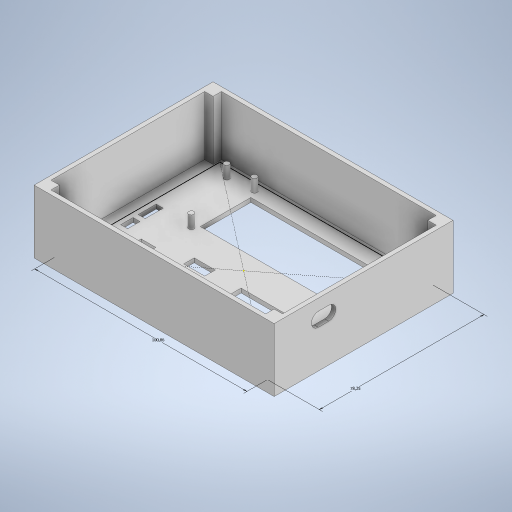
# Autodesk Inventor part: plant watner 2.0 case
Saved by Autodesk Inventor 2024 (Build 280153000, 153)
## iProperties
Created: 2024-03-16
Part Number: plant watner 2.0 case
Material: Generic
Document SubType Name: Modeling
Designer: Emil
Density: 1 g/cm^3
Appearance: Default
Author: Emil
Autodesk Inventor part; units mm, degrees
ref_plane "YZ Plane" through (0, 0, 0) normal (1, 0, 0) x (0, 1, 0)
ref_plane "XZ Plane" through (0, 0, 0) normal (0, 1, 0) x (-1, 0, 0)
ref_plane "XY Plane" through (0, 0, 0) normal (0, 0, 1) x (1, 0, 0)
sketch "Sketch1" plane through (0, 0, 0) normal (0, 1, 0) x (-1, 0, 0)
  line L0 (55, -40.5) -> (-55, -40.5)
  line L1 (-55, -40.5) -> (-55, 40.5)
  line L2 (-55, 40.5) -> (55, 40.5)
  line L3 (55, 40.5) -> (55, -40.5)
  line L4 (55, -40.5) -> (-55, 40.5) construction
  line L5 (-55, -40.5) -> (55, 40.5) construction
  line L6 (57, 42.5) -> (-57, 42.5)
  line L7 (-57, 42.5) -> (-57, -42.5)
  line L8 (-57, -42.5) -> (57, -42.5)
  line L9 (57, -42.5) -> (57, 42.5)
  line L10 (57, 42.5) -> (-57, -42.5) construction
  line L11 (-57, 42.5) -> (57, -42.5) construction
  line L12 (50.43, 39.125) -> (-50.43, 39.125)
  line L13 (-50.43, 39.125) -> (-50.43, -39.125)
  line L14 (-50.43, -39.125) -> (50.43, -39.125)
  line L15 (50.43, -39.125) -> (50.43, 39.125)
  line L16 (50.43, 39.125) -> (-50.43, -39.125) construction
  line L17 (-50.43, 39.125) -> (50.43, -39.125) construction
  point P0 (0, 0)
  dimension "d0" = 110
  dimension "d1" = 81
  dimension "d2" = 114
  dimension "d3" = 85
  dimension "d190" = 100.86
  dimension "d191" = 78.25
  constraints: 36 end point, 6 midpoint, 6 parallel, 3 horizontal, 3 perpendicular
  measures "d0" distance of L1.end L2.end
  measures "d1" distance of L0.end L1.end
  measures "d2" distance of L8.end L7.end
  measures "d3" distance of L7.end L6.end
  measures "d190" distance of L14.end L13.end
  measures "d191" distance of L14.end L12.start
extrude "Extrusion1" add sketch "Sketch1" along normal blind 30 contours L9 L8 L7 L6
sketch "Sketch2" plane through (0, 0, 0) normal (0, 1, 0) x (-1, 0, 0)
  line L0 (-55, -40.5) -> (-55, 40.5) projected
  line L1 (55, 40.5) -> (-55, 40.5)
  line L2 (-55, 40.5) -> (-55, -40.5)
  line L3 (-55, -40.5) -> (55, -40.5)
  line L4 (55, -40.5) -> (55, 40.5)
  line L5 (55, 40.5) -> (-55, -40.5) construction
  line L6 (-55, 40.5) -> (55, -40.5) construction
  point P0 (0, 0)
  constraints: 12 end point, 2 midpoint, 2 parallel, 1 horizontal, 1 perpendicular
extrude "Extrusion2" add sketch "Sketch2" along normal blind 2
sketch "Sketch3" plane through (0, 0, 0) normal (0, -1, 0) x (1, 0, 0)
  line L0 (42.57, -31.875) -> (-28.43, -31.875)
  line L1 (-28.43, -31.875) -> (-28.43, -7.875)
  line L2 (-28.43, -7.875) -> (42.57, -7.875)
  line L3 (42.57, -7.875) -> (42.57, -31.875)
  line L4 (34.53, 35.725) -> (6.53, 35.725)
  line L5 (6.53, 35.725) -> (6.53, 7.725)
  line L6 (6.53, 7.725) -> (34.53, 7.725)
  line L7 (34.53, 7.725) -> (34.53, 35.725)
  line L8 (-7.03, 11.425) -> (-17.03, 11.425)
  line L9 (-17.03, 11.425) -> (-17.03, 6.425)
  line L10 (-17.03, 6.425) -> (-7.03, 6.425)
  line L11 (-7.03, 6.425) -> (-7.03, 11.425)
  line L12 (50.43, 39.125) -> (-50.43, 39.125)
  line L13 (-50.43, 39.125) -> (-50.43, -39.125)
  line L14 (-50.43, -39.125) -> (50.43, -39.125)
  line L15 (50.43, -39.125) -> (50.43, 39.125)
  line L16 (50.43, 39.125) -> (-50.43, -39.125) construction
  line L17 (-50.43, 39.125) -> (50.43, -39.125) construction
  line L18 (-30.4304, 18.225) -> (-37.4304, 18.225)
  line L19 (-37.4304, 18.225) -> (-37.4304, 11.225)
  line L20 (-37.4304, 11.225) -> (-30.4304, 11.225)
  line L21 (-30.4304, 11.225) -> (-30.4304, 18.225)
  line L22 (-30.4304, 18.225) -> (-37.4304, 11.225) construction
  line L23 (-37.4304, 18.225) -> (-30.4304, 11.225) construction
  line L24 (-30.4304, 33.4598) -> (-37.4304, 33.4598)
  line L25 (-37.4304, 33.4598) -> (-37.4304, 26.4598)
  line L26 (-37.4304, 26.4598) -> (-30.4304, 26.4598)
  line L27 (-30.4304, 26.4598) -> (-30.4304, 33.4598)
  line L28 (-30.4304, 33.4598) -> (-37.4304, 26.4598) construction
  line L29 (-37.4304, 33.4598) -> (-30.4304, 26.4598) construction
  line L30 (-23.8133, 25.9138) -> (-30.8133, 25.9138)
  line L31 (-30.8133, 25.9138) -> (-30.8133, 18.9138)
  line L32 (-30.8133, 18.9138) -> (-23.8133, 18.9138)
  line L33 (-23.8133, 18.9138) -> (-23.8133, 25.9138)
  line L34 (-23.8133, 25.9138) -> (-30.8133, 18.9138) construction
  line L35 (-30.8133, 25.9138) -> (-23.8133, 18.9138) construction
  line L36 (-36.8875, 25.9138) -> (-43.8875, 25.9138)
  line L37 (-43.8875, 25.9138) -> (-43.8875, 18.9138)
  line L38 (-43.8875, 18.9138) -> (-36.8875, 18.9138)
  line L39 (-36.8875, 18.9138) -> (-36.8875, 25.9138)
  line L40 (-36.8875, 25.9138) -> (-43.8875, 18.9138) construction
  line L41 (-43.8875, 25.9138) -> (-36.8875, 18.9138) construction
  line L42 (-50.43, 39.125) -> (50.4731, 39.0489) construction
  line L43 (50.4731, 39.0489) -> (50.4141, -39.1891) construction
  line L44 (50.4141, -39.1891) -> (-50.489, -39.113) construction
  line L45 (-50.489, -39.113) -> (-50.43, 39.125) construction
  line L46 (17.9042, 35.3523) -> (15.6181, 35.3523)
  line L47 (47.7465, 12.6947) -> (44.5311, 12.6947)
  line L48 (46.7465, 20.4524) -> (43.1682, 20.4524)
  line L49 (-57, 42.5) -> (57, 42.5) projected
  line L50 (-44.8275, -6.6468) -> (-48.1514, -6.6468)
  line L51 (-48.1514, -6.6468) -> (-48.1514, 1.9287)
  line L52 (-48.1514, 1.9287) -> (-44.8275, 1.9287)
  line L53 (-44.8275, 1.9287) -> (-44.8275, -6.6468)
  line L54 (-44.8275, 4.375) -> (-48.1514, 4.375)
  line L55 (-48.1514, 4.375) -> (-48.1514, 10.225)
  line L56 (-48.1514, 10.225) -> (-44.8275, 10.225)
  line L57 (-44.8275, 10.225) -> (-44.8275, 4.375)
  point P0 (0, 0)
  point P1 (-33.9304, 14.725)
  point P2 (-33.9304, 29.9598)
  point P3 (-27.3133, 22.4138)
  point P4 (-40.3875, 22.4138)
  point P5 (46.1388, 12.6947)
  dimension "d8" = 71
  dimension "d9" = 24
  dimension "d18" = 28
  dimension "d19" = 28
  dimension "d20" = 10
  dimension "d21" = 5
  dimension "d22" = 100.86
  dimension "d23" = 78.25
  dimension "d31" = 3.4
  dimension "d32" = 15.9
  dimension "d33" = 22
  dimension "d35" = 33.4
  dimension "d36" = 27.7
  dimension "d45" = 7
  dimension "d46" = 7
  dimension "d47" = 7
  dimension "d48" = 7
  dimension "d135" = 7
  dimension "d136" = 7
  dimension "d137" = 7
  dimension "d138" = 7
  dimension "d203" = 47
  dimension "d580" = 3.7727
  dimension "d585" = 22.0476
  constraints: 106 end point, 21 equal length, 13 horizontal, 11 midpoint, 10 perpendicular, 3 point on line, 1 coincident, 2 other
  measures "d8" distance of L1.end L2.end
  measures "d9" distance of L0.end L1.end
  measures "d18" distance of L6.end L5.end
  measures "d19" distance of L5.end L4.end
  measures "d20" distance of L10.end L9.end
  measures "d21" distance of L9.end L8.end
  measures "d22" distance of L14.end L13.end
  measures "d23" distance of L13.end L12.end
  measures "d31" distance between parallel lines of L12 L4
  measures "d32" distance between parallel lines of L15 L7
  measures "d33" distance between parallel lines of L13 L1
  measures "d35" distance between parallel lines of L13 L9
  measures "d36" distance between parallel lines of L12 L8
  measures "d45" distance of L20.end L19.end
  measures "d46" distance of L19.end L18.end
  measures "d47" distance of L27.start L26.start
  measures "d48" distance of L26.start L24.end
  measures "d135" distance of L32.end L31.end
  measures "d136" distance of L31.end L30.end
  measures "d137" distance of L38.end L37.end
  measures "d138" distance of L37.end L36.end
  measures "d203" distance between parallel lines of L2 L12
  measures "d580" distance between parallel lines of L12 L46
  measures "d585" distance between parallel lines of L49 L48
extrude "Extrusion3" cut sketch "Sketch3" against normal blind 30 contours L0 L1 L2 L3 | L7 L6 L5 L4 | L11 L10 L9 L8 | L21 L20 L19 L18 | L27 L26 L25 L24 | L33 L32 L31 L30 | L39 L38 L37 L36 | L50 L51 L52 L53 | L54 L55 L56 L57
sketch "Sketch4" plane through (0, 2, 0) normal (0, 1, 0) x (1, 0, 0)
  circle A0 centre (-45.13, -34.025) radius 1.25
  line L0 (55, -40.5) -> (-55, -40.5) projected
  line L1 (-55, -40.5) -> (-55, 40.5) projected
  circle A1 centre (-42.23, 34.175) radius 1.25
  line L2 (-55, 40.5) -> (55, 40.5) projected
  circle A2 centre (45.31, -34.725) radius 1.25
  line L3 (55, 40.5) -> (55, -40.5) projected
  line L4 (-50.43, -39.125) -> (50.43, -39.125)
  line L5 (50.43, -39.125) -> (50.43, 39.125)
  line L6 (50.43, 39.125) -> (-50.43, 39.125)
  line L7 (-50.43, 39.125) -> (-50.43, -39.125)
  line L8 (-50.43, -39.125) -> (50.43, 39.125) construction
  line L9 (50.43, -39.125) -> (-50.43, 39.125) construction
  circle A3 centre (-30.23, 35.375) radius 1.25
  circle A4 centre (44.37, 35.375) radius 1.25
  circle A5 centre (-30.23, 5.375) radius 1.25
  circle A6 centre (44.37, 5.375) radius 1.25
  line L10 (-28.43, 7.875) -> (-28.43, 31.875) projected
  line L11 (42.57, 31.875) -> (42.57, 7.875) projected
  line L12 (-28.43, 31.875) -> (42.57, 31.875) projected
  line L13 (42.57, 7.875) -> (-28.43, 7.875) projected
  line L14 (-50.43, 39.125) -> (50.4734, 39.0562) construction
  line L15 (50.4734, 39.0562) -> (50.42, -39.1821) construction
  line L16 (50.42, -39.1821) -> (-50.4834, -39.1133) construction
  line L17 (-50.4834, -39.1133) -> (-50.43, 39.125) construction
  point P0 (0, 0)
  dimension "d181" = 2.5
  dimension "d184" = 2.5
  dimension "d187" = 2.5
  dimension "d192" = 100.86
  dimension "d193" = 78.25
  dimension "d194" = 8.2
  dimension "d195" = 4.95
  dimension "d196" = 5.3
  dimension "d197" = 5.1
  dimension "d198" = 5.12
  dimension "d199" = 4.4
  dimension "d204" = 2.5
  dimension "d205" = 2.5
  dimension "d206" = 2.5
  dimension "d207" = 2.5
  dimension "d209" = 1.8
  dimension "d211" = 1.8
  dimension "d212" = 1.8
  dimension "d213" = 1.8
  dimension "d214" = 3.5
  dimension "d215" = 3.5
  dimension "d216" = 2.5
  dimension "d217" = 2.5
  constraints: 12 end point, 7 centre point, 2 midpoint, 2 parallel, 1 coincident, 1 horizontal, 1 perpendicular, 2 other
  measures "d181" diameter of A0
  measures "d184" diameter of A1
  measures "d187" diameter of A2
  measures "d192" distance of L6.end L5.end
  measures "d193" distance of L6.end L4.start
  measures "d194" distance from line of A1.centre L7
  measures "d195" distance from line of A1.centre L6
  measures "d196" distance from line of A0.centre L7
  measures "d197" distance from line of A0.centre L4
  measures "d198" distance from line of A2.centre L5
  measures "d199" distance from line of A2.centre L4
  measures "d204" diameter of A3
  measures "d205" diameter of A4
  measures "d206" diameter of A5
  measures "d207" diameter of A6
  measures "d209" distance from line of L10 A3.centre
  measures "d211" distance from line of L11 A4.centre
  measures "d212" distance from line of L10 A5.centre
  measures "d213" distance from line of L11 A6.centre
  measures "d214" distance from line of L12 A3.centre
  measures "d215" distance from line of L12 A4.centre
  measures "d216" distance from line of L13 A5.centre
  measures "d217" distance from line of L13 A6.centre
extrude "Extrusion4" add sketch "Sketch4" along normal blind 6 contours A0 | A1 | A2 | A3 | A4 | A5 | A6
sketch "Sketch5" plane through (0, 2, 0) normal (0, 1, 0) x (1, 0, 0)
  line L0 (50.43, 39.125) -> (-50.43, 39.125)
  line L1 (-50.43, 39.125) -> (-50.43, -39.125)
  line L2 (-50.43, -39.125) -> (50.43, -39.125)
  line L3 (50.43, -39.125) -> (50.43, 39.125)
  line L4 (50.43, 39.125) -> (-50.43, -39.125) construction
  line L5 (-50.43, 39.125) -> (50.43, -39.125) construction
  point P0 (0, 0)
  dimension "d352" = 78.25
  dimension "d353" = 100.86
  constraints: 12 end point, 2 midpoint, 2 parallel, 1 horizontal, 1 perpendicular
  measures "d352" distance of L2.end L0.start
  measures "d353" distance of L1.end L2.end
sketch "Sketch6" plane through (0, 2, 0) normal (0, 1, 0) x (1, 0, 0)
  line L0 (55, -40.5) -> (-55, -40.5) projected
  line L1 (55, -40.5) -> (51, -40.5)
  line L2 (51, -40.5) -> (51, -36.5)
  line L3 (51, -36.5) -> (55, -36.5)
  line L4 (55, -36.5) -> (55, -40.5)
  line L5 (-55, 40.5) -> (55, 40.5) projected
  line L6 (55, 40.5) -> (51, 40.5)
  line L7 (51, 40.5) -> (51, 36.5)
  line L8 (51, 36.5) -> (55, 36.5)
  line L9 (55, 36.5) -> (55, 40.5)
  line L10 (-54.9902, -40.5) -> (-50.9902, -40.5)
  line L11 (-50.9902, -40.5) -> (-50.9902, -36.5)
  line L12 (-50.9902, -36.5) -> (-54.9902, -36.5)
  line L13 (-54.9902, -36.5) -> (-55, -36.5)
  line L14 (55, -40.5) -> (-55, -40.5) projected
  line L15 (-50.9902, -40.5) -> (-55, -40.5)
  line L16 (-55, -40.5) -> (-55, -36.5)
  line L17 (-55, 40.5) -> (55, 40.5) projected
  line L18 (-50.424, 39.0879) -> (50.4561, 39.0879) construction
  line L19 (50.4561, 39.0879) -> (50.4561, -39.1323) construction
  line L20 (50.4561, -39.1323) -> (-50.424, -39.1323) construction
  line L21 (-50.424, -39.1323) -> (-50.424, 39.0879) construction
  line L22 (-49.2051, 39.0879) -> (-45.6234, 39.0879)
  line L23 (-48.1397, 6.687) -> (-44.6458, 6.687)
  line L24 (-48.2072, -10.3595) -> (-44.6458, -10.3595)
  line L25 (-55, 40.5) -> (-51, 40.5)
  line L26 (-51, 40.5) -> (-51, 36.5)
  line L27 (-51, 36.5) -> (-55, 36.5)
  line L28 (-55, 36.5) -> (-55, 40.5)
  line L29 (-51, 40.5) -> (51, 40.5)
  line L30 (57, 42.5) -> (-57, 42.5) projected
  line L31 (55, 36.5) -> (55, -36.5)
  line L32 (51, -40.5) -> (-50.9902, -40.5)
  line L33 (-55, -36.5) -> (-55, 36.5)
  line L34 (55, 40.5) -> (55, -40.5) projected
  line L35 (55, 40.5) -> (55, -40.5)
  line L36 (55, 40.5) -> (55, -40.5)
  point P0 (0, 0)
  dimension "d443" = 4
  dimension "d444" = 4
  dimension "d445" = 4
  dimension "d446" = 4
  dimension "d447" = 4
  dimension "d448" = 4
  dimension "d564" = 30.1405
  dimension "d591" = 4
  dimension "d592" = 4
  dimension "d599" = 110
  dimension "d600" = 81
  constraints: 54 end point, 8 horizontal, 8 parallel, 7 perpendicular, 3 collinear, 3 point on line, 2 other
  measures "d443" distance of L2.end L3.end
  measures "d444" distance of L1.end L2.end
  measures "d445" distance of L8.end L7.end
  measures "d446" distance of L7.end L6.end
  measures "d447" distance of L12.end L11.end
  measures "d448" distance of L11.end L10.end
  measures "d564" distance between parallel lines of L0 L24
  measures "d591" distance of L26.end L27.end
  measures "d592" distance of L25.end L26.end
  measures "d599" distance of L5.start L5.end
  measures "d600" distance of L5.end L0.start
extrude "Extrusion5" add sketch "Sketch6" along normal up to surface (28 mm away) contours L0 L2 L3 L4 | L0 L16 L13 L12 L11 | L8 L7 L5 L9 | L26 L27 L28 L5
sketch "Sketch8" plane through (57, 0, 42.5) normal (1, 0, 0) x (0, 0, -1)
  line L0 (26, 24.5926) -> (26, 18) construction
  line L1 (26, 24.5926) -> (32.5926, 24.5926) construction
  line L2 (26, 18) -> (21, 18)
  line L3 (21, 18) -> (22.6917, 18)
  line L4 (26, 24.5926) -> (21, 24.5926)
  arc A0 (21, 24.5926) -> (21, 18) centre (21, 21.2963) ccw
  arc A1 (26, 18) -> (26, 24.5926) centre (26, 21.2963) ccw
  line L5 (0, 30) -> (85, 30) projected
  line L6 (0, 0) -> (0, 30) projected
  line L7 (0, 0) -> (85, 0) projected
  point P0 (42.5, 0)
  point P1 (0, 15)
  point P2 (17.7037, 21.2963)
  dimension "d573" = 90
  dimension "d574" = 5
  dimension "d578" = 18
  dimension "d579" = 21
  dimension "d586" = 17.7037
  constraints: 10 end point, 5 point on circle, 3 tangent, 2 centre point, 2 horizontal, 2 point on line, 1 midpoint, 1 perpendicular
  measures "d573" angle of L0 L1
  measures "d574" distance of L0.end L2.end
  measures "d578" distance from line of L7 L2.end
  measures "d579" distance from line of L6 L2.end
  measures "d586" distance from line of L6 point (17.704, 21.296)
extrude "Extrusion9" cut sketch "Sketch8" against normal blind 3
body "Solid1"
